Autodesk Inventor part; units mm, degrees
note: some values were not read from the file. Chosen so that the rebuilt part matches the saved one: direction of "Hole2".
(part 4 of 20)
  ellipse E392 centre (-10072.326927, -10029.332215) end of major axis (-10072.501043, -10029.408266) minor radius 0.168992 (-10072.321099, -10029.159944) -> (-10072.360635, -10029.165817) ccw
  ellipse E393 centre (-10070.302682, -10029.229876) end of major axis (-10070.476798, -10029.305926) minor radius 0.168992 (-10070.177973, -10029.092016) -> (-10070.296853, -10029.057605) ccw
  ellipse E394 centre (-10070.177499, -10030.249171) end of major axis (-10070.36739, -10030.242746) minor radius 0.079929 (-10070.142738, -10030.328755) -> (-10070.027446, -10030.302364) ccw
  ellipse E395 centre (-10072.201744, -10030.35151) end of major axis (-10072.391636, -10030.345086) minor radius 0.079929 (-10072.388447, -10030.360949) -> (-10072.166984, -10030.431094) ccw
  line L492 (-10072.72794, -10030.167115) -> (-10074.103641, -10030.236666)
  line L493 (-10074.255583, -10030.325688) -> (-10073.85675, -10031.238806)
  line L494 (-10067.96089, -10030.940729) -> (-10068.359722, -10030.027612)
  line L495 (-10068.581185, -10029.957468) -> (-10069.956886, -10030.027019)
  line L496 (-10072.723339, -10030.031111) -> (-10074.09904, -10030.100662)
  line L497 (-10068.576584, -10029.821464) -> (-10069.952284, -10029.891015)
  line L498 (-10067.956288, -10030.804726) -> (-10068.355121, -10029.891609)
  ellipse E396 centre (-10074.06888, -10030.316249) end of major axis (-10074.258772, -10030.309825) minor radius 0.079929 (-10074.103641, -10030.236666) -> (-10074.255583, -10030.325688) ccw
  ellipse E397 centre (-10068.546425, -10030.037051) end of major axis (-10068.356533, -10030.043476) minor radius 0.079929 (-10068.359722, -10030.027612) -> (-10068.581185, -10029.957468) ccw
  ellipse E398 centre (-10074.064279, -10030.180246) end of major axis (-10074.25417, -10030.173821) minor radius 0.079929 (-10074.09904, -10030.100662) -> (-10074.25417, -10030.173821) ccw
  ellipse E399 centre (-10068.541823, -10029.901048) end of major axis (-10068.351932, -10029.907472) minor radius 0.079929 (-10068.355121, -10029.891609) -> (-10068.576584, -10029.821464) ccw
  line L499 (-10074.258772, -10030.309825) -> (-10074.25417, -10030.173821)
  line L500 (-10067.871011, -10029.740777) -> (-10067.902882, -10030.682769)
  line L501 (-10067.875439, -10030.745598) -> (-10067.841392, -10029.73928)
  ellipse E400 centre (-10067.948619, -10030.578053) end of major axis (-10067.935996, -10030.827734) minor radius 0.044682 (-10067.956288, -10030.804726) -> (-10067.902882, -10030.682769) ccw
  ellipse E401 centre (-10073.84448, -10030.876129) end of major axis (-10073.824283, -10031.275619) minor radius 0.071491 (-10073.85675, -10031.238806) -> (-10073.824283, -10031.275619) ccw
  ellipse E402 centre (-10067.948619, -10030.578053) end of major axis (-10067.928422, -10030.977543) minor radius 0.071491 (-10067.96089, -10030.940729) -> (-10067.875439, -10030.745598) ccw
  line L502 (-10073.824283, -10031.275619) -> (-10072.075178, -10031.18719)
  line L503 (-10069.677528, -10031.065972) -> (-10067.928422, -10030.977543)
  ellipse E403 centre (-10072.802697, -10009.479709) end of major axis (-10072.614174, -10009.456065) minor radius 0.095931 (-10072.613936, -10009.458421) -> (-10072.809979, -10009.383969) ccw
  line L504 (-10072.614174, -10009.456065) -> (-10072.610843, -10009.482618)
  line L505 (-10072.598783, -10009.657643) -> (-10072.613936, -10009.458421)
  line L506 (-10070.180999, -10009.3015) -> (-10070.166094, -10009.497453)
  line L507 (-10070.347572, -10009.614481) -> (-10071.235682, -10009.714641)
  line L508 (-10072.809979, -10009.383969) -> (-10074.200844, -10009.540829)
  line L509 (-10074.382322, -10009.657857) -> (-10074.366628, -10009.864192)
  line L510 (-10068.337917, -10010.084094) -> (-10068.409482, -10009.143227)
  line L511 (-10068.326139, -10010.155581) -> (-10068.374133, -10009.524607)
  ellipse E404 centre (-10074.193562, -10009.636569) end of major axis (-10074.382085, -10009.660213) minor radius 0.095931 (-10074.200844, -10009.540829) -> (-10074.382322, -10009.657857) ccw
  ellipse E405 centre (-10070.354854, -10009.518741) end of major axis (-10070.166331, -10009.495097) minor radius 0.095931 (-10070.347572, -10009.614481) -> (-10070.166094, -10009.497453) ccw
  ellipse E406 centre (-10068.294951, -10010.426681) end of major axis (-10068.250123, -10010.824161) minor radius 0.00852 (-10068.337917, -10010.084094) -> (-10068.331861, -10010.154713) ccw
  line L512 (-10074.363014, -10028.330212) -> (-10074.369736, -10028.432806)
  line L513 (-10068.399185, -10028.956994) -> (-10068.349903, -10028.204791)
  line L514 (-10068.533523, -10028.105039) -> (-10068.666725, -10028.090017)
  line L515 (-10068.370793, -10028.641723) -> (-10068.333284, -10028.069217)
  line L516 (-10072.60135, -10028.632241) -> (-10072.595095, -10028.536769)
  line L517 (-10071.184925, -10028.471649) -> (-10070.345198, -10028.566352)
  line L518 (-10070.161579, -10028.666104) -> (-10070.177271, -10028.905625)
  ellipse E407 centre (-10072.557033, -10028.27071) end of major axis (-10072.60186, -10028.668191) minor radius 0.00852 (-10072.60135, -10028.632241) -> (-10072.602641, -10028.659347) ccw
  ellipse E408 centre (-10070.132954, -10028.544094) end of major axis (-10070.177781, -10028.941574) minor radius 0.00852 (-10070.177271, -10028.905625) -> (-10070.177781, -10028.941574) ccw
  ellipse E409 centre (-10070.350339, -10028.644816) end of major axis (-10070.16175, -10028.667933) minor radius 0.078528 (-10070.161579, -10028.666104) -> (-10070.345198, -10028.566352) ccw
  ellipse E410 centre (-10068.538663, -10028.183503) end of major axis (-10068.350075, -10028.206621) minor radius 0.078528 (-10068.349903, -10028.204791) -> (-10068.533523, -10028.105039) ccw
  ellipse E411 centre (-10068.522044, -10028.047929) end of major axis (-10068.333456, -10028.071046) minor radius 0.078528 (-10068.333284, -10028.069217) -> (-10068.343012, -10028.040958) ccw
  ellipse E412 centre (-10074.325419, -10028.071275) end of major axis (-10074.370246, -10028.468755) minor radius 0.00852 (-10074.369736, -10028.432806) -> (-10074.370246, -10028.468755) ccw
  line L519 (-10074.370246, -10028.468755) -> (-10074.342698, -10028.471862)
  line L520 (-10070.177781, -10028.941574) -> (-10070.167273, -10028.942759)
  ellipse E413 centre (-10072.246386, -10007.126413) end of major axis (-10072.067085, -10007.189273) minor radius 0.159857 (-10072.059684, -10007.135852) -> (-10072.10068, -10007.038353) ccw
  ellipse E414 centre (-10072.273208, -10007.202921) end of major axis (-10072.093908, -10007.265781) minor radius 0.159857 (-10072.086506, -10007.21236) -> (-10072.121744, -10007.121966) ccw
  ellipse E415 centre (-10072.289789, -10007.05931) end of major axis (-10072.100103, -10007.048406) minor radius 0.096916 (-10072.103087, -10007.068749) -> (-10072.100103, -10007.048406) ccw
  ellipse E416 centre (-10072.297194, -10006.930504) end of major axis (-10072.107507, -10006.9196) minor radius 0.096916 (-10072.110492, -10006.939943) -> (-10072.263219, -10006.833594) ccw
  ellipse E417 centre (-10069.52614, -10007.0706) end of major axis (-10069.715826, -10007.081504) minor radius 0.096916 (-10069.492164, -10006.97369) -> (-10069.712842, -10007.061161) ccw
  line L521 (-10072.107507, -10006.9196) -> (-10072.100103, -10007.048406)
  line L522 (-10072.081203, -10007.304616) -> (-10072.086506, -10007.21236)
  line L523 (-10072.059684, -10007.135852) -> (-10072.047289, -10007.35146)
  line L524 (-10072.221358, -10007.256177) -> (-10072.110492, -10006.939943)
  line L525 (-10072.103087, -10007.068749) -> (-10072.19317, -10007.3257)
  line L526 (-10072.500311, -10008.05186) -> (-10072.396598, -10007.756029)
  line L527 (-10072.17592, -10007.668558) -> (-10070.151675, -10007.770897)
  line L528 (-10069.998948, -10007.877247) -> (-10070.102661, -10008.173078)
  line L529 (-10069.712842, -10007.061161) -> (-10069.823708, -10007.377394)
  line L530 (-10070.044385, -10007.464865) -> (-10072.068631, -10007.362526)
  ellipse E418 centre (-10072.480566, -10008.395343) end of major axis (-10072.460369, -10007.995853) minor radius 0.071491 (-10072.500311, -10008.05186) -> (-10072.554705, -10008.484751) ccw
  ellipse E419 centre (-10072.480566, -10008.395343) end of major axis (-10072.493189, -10008.645024) minor radius 0.044682 (-10072.492906, -10008.180666) -> (-10072.525255, -10008.39437) ccw
  line L531 (-10072.389193, -10007.884835) -> (-10072.492906, -10008.180666)
  ellipse E420 centre (-10070.082916, -10008.51656) end of major axis (-10070.103113, -10008.91605) minor radius 0.071491 (-10070.102661, -10008.173078) -> (-10070.157073, -10008.608429) ccw
  line L532 (-10070.14427, -10007.899703) -> (-10072.168516, -10007.797364)
  line L533 (-10070.358201, -10009.301066) -> (-10070.663673, -10009.285622)
  line L534 (-10071.882761, -10009.223989) -> (-10072.312978, -10009.202239)
  line L535 (-10067.939751, -10007.422007) -> (-10067.880499, -10008.452725)
  line L536 (-10067.849188, -10008.454308) -> (-10067.912929, -10007.345499)
  ellipse E421 centre (-10068.126453, -10007.412568) end of major axis (-10067.947153, -10007.475428) minor radius 0.159857 (-10067.939751, -10007.422007) -> (-10067.974989, -10007.331613) ccw
  ellipse E422 centre (-10068.099631, -10007.33606) end of major axis (-10067.92033, -10007.39892) minor radius 0.159857 (-10067.912929, -10007.345499) -> (-10067.953925, -10007.248) ccw
  line L537 (-10072.263219, -10006.833594) -> (-10073.63892, -10006.764043)
  line L538 (-10073.859597, -10006.851514) -> (-10074.249416, -10007.963431)
  line L539 (-10068.353556, -10008.261507) -> (-10067.963737, -10007.14959)
  line L540 (-10068.116464, -10007.043241) -> (-10069.492164, -10006.97369)
  line L541 (-10068.346151, -10008.390313) -> (-10067.956332, -10007.278396)
  ellipse E423 centre (-10073.672895, -10006.860953) end of major axis (-10073.862581, -10006.871858) minor radius 0.096916 (-10073.63892, -10006.764043) -> (-10073.859597, -10006.851514) ccw
  ellipse E424 centre (-10068.150439, -10007.140151) end of major axis (-10067.960752, -10007.129247) minor radius 0.096916 (-10067.963737, -10007.14959) -> (-10068.116464, -10007.043241) ccw
  ellipse E425 centre (-10068.143034, -10007.268957) end of major axis (-10067.953347, -10007.258053) minor radius 0.096916 (-10067.956332, -10007.278396) -> (-10067.953347, -10007.258053) ccw
  line L542 (-10067.960752, -10007.129247) -> (-10067.953347, -10007.258053)
  ellipse E426 centre (-10072.209895, -10007.765468) end of major axis (-10072.399582, -10007.776372) minor radius 0.096916 (-10072.17592, -10007.668558) -> (-10072.396598, -10007.756029) ccw
  ellipse E427 centre (-10070.18565, -10007.867808) end of major axis (-10069.995963, -10007.856903) minor radius 0.096916 (-10069.998948, -10007.877247) -> (-10070.151675, -10007.770897) ccw
  ellipse E428 centre (-10070.01041, -10007.367955) end of major axis (-10069.820723, -10007.357051) minor radius 0.096916 (-10070.044385, -10007.464865) -> (-10069.823708, -10007.377394) ccw
  ellipse E429 centre (-10072.034655, -10007.265616) end of major axis (-10072.224342, -10007.27652) minor radius 0.096916 (-10072.221358, -10007.256177) -> (-10072.068631, -10007.362526) ccw
  ellipse E430 centre (-10072.202491, -10007.894274) end of major axis (-10072.392178, -10007.905178) minor radius 0.096916 (-10072.168516, -10007.797364) -> (-10072.389193, -10007.884835) ccw
  ellipse E431 centre (-10072.313886, -10008.961649) end of major axis (-10072.493186, -10008.898789) minor radius 0.159857 (-10072.33531, -10009.121035) -> (-10072.324798, -10009.122819) ccw
  ellipse E432 centre (-10072.340708, -10009.038157) end of major axis (-10072.161408, -10009.101016) minor radius 0.159857 (-10072.363459, -10009.197281) -> (-10072.348281, -10009.199785) ccw
  ellipse E433 centre (-10070.316463, -10009.140496) end of major axis (-10070.137162, -10009.203356) minor radius 0.159857 (-10070.251159, -10009.298888) -> (-10070.185446, -10009.268734) ccw
  ellipse E434 centre (-10070.28964, -10009.063988) end of major axis (-10070.468941, -10009.001128) minor radius 0.159857 (-10070.236148, -10009.224709) -> (-10070.189719, -10009.210719) ccw
  ellipse E435 centre (-10070.178245, -10007.996614) end of major axis (-10069.988559, -10007.985709) minor radius 0.096916 (-10070.019731, -10007.936529) -> (-10070.14427, -10007.899703) ccw
  line L543 (-10068.338763, -10009.424007) -> (-10068.374927, -10008.794905)
  line L544 (-10068.400279, -10008.897002) -> (-10068.388749, -10009.097559)
  line L545 (-10068.3686, -10009.448068) -> (-10068.365318, -10009.505168)
  ellipse E436 centre (-10068.33381, -10008.60499) end of major axis (-10068.321187, -10008.355308) minor radius 0.044682 (-10068.346151, -10008.390313) -> (-10068.371921, -10008.521801) ccw
  ellipse E437 centre (-10074.229671, -10008.306913) end of major axis (-10074.249868, -10008.706403) minor radius 0.071491 (-10074.249416, -10007.963431) -> (-10074.303499, -10008.450252) ccw
  ellipse E438 centre (-10068.33381, -10008.60499) end of major axis (-10068.354007, -10009.004479) minor radius 0.071491 (-10068.353556, -10008.261507) -> (-10068.4065, -10008.630689) ccw
  ellipse E439 centre (-10072.776909, -10029.133016) end of major axis (-10072.596108, -10029.074614) minor radius 0.167961 (-10072.789107, -10029.303177) -> (-10072.589277, -10029.13178) ccw
  ellipse E440 centre (-10072.755355, -10029.199743) end of major axis (-10072.574553, -10029.141341) minor radius 0.167961 (-10072.644451, -10029.32956) -> (-10072.567723, -10029.198507) ccw
  ellipse E441 centre (-10069.970499, -10029.181393) end of major axis (-10070.1513, -10029.239795) minor radius 0.167961 (-10070.1513, -10029.239795) -> (-10070.111114, -10029.303245) ccw
  ellipse E442 centre (-10072.761869, -10029.388593) end of major axis (-10072.572355, -10029.402178) minor radius 0.083645 (-10072.574237, -10029.387357) -> (-10072.789171, -10029.304073) ccw
  ellipse E443 centre (-10072.771499, -10029.522931) end of major axis (-10072.581985, -10029.536516) minor radius 0.083645 (-10072.583867, -10029.521695) -> (-10072.798801, -10029.43841) ccw
  ellipse E444 centre (-10069.986643, -10029.50458) end of major axis (-10070.176156, -10029.490995) minor radius 0.083645 (-10070.013945, -10029.42006) -> (-10070.174275, -10029.505817) ccw
  ellipse E445 centre (-10069.992053, -10029.114666) end of major axis (-10070.172854, -10029.173068) minor radius 0.167961 (-10070.179685, -10029.115902) -> (-10070.004251, -10029.284827) ccw
  ellipse E446 centre (-10069.977013, -10029.370243) end of major axis (-10070.166527, -10029.356658) minor radius 0.083645 (-10070.004315, -10029.285722) -> (-10070.166527, -10029.356658) ccw
  line L546 (-10070.172854, -10029.173068) -> (-10070.1513, -10029.239795)
  line L547 (-10070.166527, -10029.356658) -> (-10070.176156, -10029.490995)
  line L548 (-10072.531836, -10028.697875) -> (-10072.567723, -10029.198507)
  line L549 (-10072.589277, -10029.13178) -> (-10072.55339, -10028.631149)
  line L550 (-10072.494777, -10029.797499) -> (-10072.499038, -10029.784308)
  line L551 (-10072.49947, -10029.782969) -> (-10072.583867, -10029.521695)
  line L552 (-10072.574237, -10029.387357) -> (-10072.519259, -10029.557556)
  line L553 (-10070.174275, -10029.505817) -> (-10070.124475, -10029.659985)
  line L554 (-10070.245515, -10029.867378) -> (-10071.514069, -10029.875737)
  line L555 (-10071.955355, -10029.878645) -> (-10072.279843, -10029.880783)
  line L556 (-10070.161258, -10028.858843) -> (-10070.179685, -10029.115902)
  line L557 (-10072.270213, -10029.746445) -> (-10072.013835, -10029.744756)
  line L558 (-10070.580502, -10029.735311) -> (-10070.235885, -10029.73304)
  ellipse E447 centre (-10074.137908, -10029.208853) end of major axis (-10074.318709, -10029.267256) minor radius 0.167961 (-10074.318709, -10029.267256) -> (-10074.278523, -10029.330706) ccw
  ellipse E448 centre (-10068.587946, -10029.172282) end of major axis (-10068.407145, -10029.11388) minor radius 0.167961 (-10068.477042, -10029.3021) -> (-10068.400314, -10029.171046) ccw
  ellipse E449 centre (-10068.6095, -10029.105556) end of major axis (-10068.428699, -10029.047153) minor radius 0.167961 (-10068.621698, -10029.275716) -> (-10068.421868, -10029.104319) ccw
  ellipse E450 centre (-10074.159462, -10029.142127) end of major axis (-10074.340263, -10029.200529) minor radius 0.167961 (-10074.347094, -10029.143363) -> (-10074.171659, -10029.312287) ccw
  line L559 (-10074.318709, -10029.267256) -> (-10074.340263, -10029.200529)
  line L560 (-10068.400314, -10029.171046) -> (-10068.38691, -10028.984061)
  line L561 (-10068.368215, -10028.723256) -> (-10068.3415, -10028.350584)
  line L562 (-10068.621698, -10029.275716) -> (-10070.004251, -10029.284827)
  line L563 (-10068.409198, -10028.927568) -> (-10068.421868, -10029.104319)
  line L564 (-10074.347094, -10029.143363) -> (-10074.314985, -10028.695444)
  line L565 (-10072.789107, -10029.303177) -> (-10074.171659, -10029.312287)
  ellipse E451 centre (-10072.344204, -10028.696639) end of major axis (-10072.525005, -10028.755041) minor radius 0.167961 (-10072.437227, -10028.555214) -> (-10072.531836, -10028.697875) ccw
  ellipse E452 centre (-10070.272817, -10029.782857) end of major axis (-10070.083303, -10029.796442) minor radius 0.083645 (-10070.245515, -10029.867378) -> (-10070.155633, -10029.855516) ccw
  ellipse E453 centre (-10072.307144, -10029.796262) end of major axis (-10072.496658, -10029.782677) minor radius 0.083645 (-10072.494777, -10029.797499) -> (-10072.487277, -10029.812028) ccw
  ellipse E454 centre (-10072.307144, -10029.796262) end of major axis (-10072.117631, -10029.809847) minor radius 0.083645 (-10072.356839, -10029.874281) -> (-10072.279843, -10029.880783) ccw
  ellipse E455 centre (-10072.365758, -10028.629912) end of major axis (-10072.546559, -10028.688315) minor radius 0.167961 (-10072.539173, -10028.57563) -> (-10072.55339, -10028.631149) ccw
  ellipse E456 centre (-10070.263187, -10029.64852) end of major axis (-10070.452701, -10029.634935) minor radius 0.083645 (-10070.235885, -10029.73304) -> (-10070.172132, -10029.727297) ccw
  ellipse E457 centre (-10072.297515, -10029.661925) end of major axis (-10072.487028, -10029.64834) minor radius 0.083645 (-10072.347313, -10029.739925) -> (-10072.270213, -10029.746445) ccw
  line L566 (-10072.798801, -10029.43841) -> (-10074.181353, -10029.447521)
  line L567 (-10074.341684, -10029.533278) -> (-10074.268765, -10029.759019)
  line L568 (-10068.300338, -10029.853716) -> (-10068.416458, -10029.494234)
  line L569 (-10068.631392, -10029.41095) -> (-10070.013945, -10029.42006)
  line L570 (-10072.789171, -10029.304073) -> (-10074.171724, -10029.313183)
  line L571 (-10068.621762, -10029.276612) -> (-10070.004315, -10029.285722)
  line L572 (-10068.093576, -10030.329659) -> (-10068.406828, -10029.359896)
  ellipse E458 centre (-10074.154052, -10029.532041) end of major axis (-10074.343565, -10029.518456) minor radius 0.083645 (-10074.181353, -10029.447521) -> (-10074.341684, -10029.533278) ccw
  ellipse E459 centre (-10068.60409, -10029.49547) end of major axis (-10068.414576, -10029.509055) minor radius 0.083645 (-10068.416458, -10029.494234) -> (-10068.631392, -10029.41095) ccw
  ellipse E460 centre (-10074.144422, -10029.397704) end of major axis (-10074.333936, -10029.384119) minor radius 0.083645 (-10074.171724, -10029.313183) -> (-10074.333936, -10029.384119) ccw
  ellipse E461 centre (-10068.59446, -10029.361133) end of major axis (-10068.404946, -10029.374718) minor radius 0.083645 (-10068.406828, -10029.359896) -> (-10068.621762, -10029.276612) ccw
  line L573 (-10074.343565, -10029.518456) -> (-10074.333936, -10029.384119)
  line L574 (-10068.032803, -10030.094217) -> (-10068.041603, -10030.216974)
  line L575 (-10068.020049, -10030.283701) -> (-10068.004197, -10030.062566)
  ellipse E462 centre (-10068.077526, -10030.105763) end of major axis (-10068.075879, -10030.355758) minor radius 0.039312 (-10068.093576, -10030.329659) -> (-10068.041603, -10030.216974) ccw
  ellipse E463 centre (-10068.077526, -10030.105763) end of major axis (-10068.080162, -10029.705772) minor radius 0.062899 (-10068.046247, -10030.460713) -> (-10068.020049, -10030.283701) ccw
  line L576 (-10072.577571, -10009.532359) -> (-10072.577053, -10009.432226)
  line L577 (-10072.560025, -10009.540558) -> (-10072.560176, -10009.569905)
  line L578 (-10070.342414, -10009.407096) -> (-10072.389265, -10009.607054)
  ellipse E464 centre (-10074.155851, -10009.382773) end of major axis (-10074.344261, -10009.407304) minor radius 0.092496 (-10074.341028, -10009.382975) -> (-10074.344639, -10009.401215) ccw
  ellipse E465 centre (-10068.554808, -10008.967185) end of major axis (-10068.366398, -10008.942654) minor radius 0.092496 (-10068.366021, -10008.948742) -> (-10068.366398, -10008.942654) ccw
  line L579 (-10068.366462, -10008.942166) -> (-10068.366398, -10008.942654)
  line L580 (-10074.344639, -10009.401215) -> (-10074.344914, -10009.454519)
  line L581 (-10068.385879, -10009.388256) -> (-10068.384314, -10009.085206)
  line L582 (-10068.369231, -10009.57016) -> (-10068.367254, -10009.187466)
  line L583 (-10068.366026, -10008.949747) -> (-10068.366021, -10008.948742)
  ellipse E466 centre (-10070.341933, -10009.313958) end of major axis (-10070.153523, -10009.289427) minor radius 0.092496 (-10070.342414, -10009.407096) -> (-10070.179086, -10009.34494) ccw
  ellipse E467 centre (-10072.388783, -10009.513916) end of major axis (-10072.577193, -10009.538448) minor radius 0.092496 (-10072.577571, -10009.532359) -> (-10072.389265, -10009.607054) ccw
  line L584 (-10074.342817, -10028.466107) -> (-10074.337905, -10028.703084)
  line L585 (-10068.381381, -10029.035724) -> (-10068.386397, -10028.79374)
  line L586 (-10068.363977, -10028.927724) -> (-10068.369259, -10028.672848)
  line L587 (-10072.571652, -10028.760795) -> (-10072.574544, -10028.621296)
  line L588 (-10071.996094, -10028.594581) -> (-10070.340635, -10028.756304)
  line L589 (-10072.555629, -10028.586144) -> (-10072.554791, -10028.62657)
  ellipse E468 centre (-10072.385757, -10028.639739) end of major axis (-10072.574269, -10028.61601) minor radius 0.082693 (-10072.442527, -10028.554595) -> (-10072.574544, -10028.621296) ccw
  ellipse E469 centre (-10070.338906, -10028.839697) end of major axis (-10070.527419, -10028.815968) minor radius 0.082693 (-10070.171544, -10028.818209) -> (-10070.340635, -10028.756304) ccw
  ellipse E470 centre (-10074.292929, -10028.345775) end of major axis (-10074.33182, -10028.74388) minor radius 0.022991 (-10074.337905, -10028.703084) -> (-10074.33182, -10028.74388) ccw
  line L590 (-10074.33182, -10028.74388) -> (-10074.31855, -10028.745177)
  line L591 (-10068.066947, -10007.915921) -> (-10068.053326, -10008.079123)
  line L592 (-10068.026512, -10008.074856) -> (-10068.045991, -10007.841482)
  ellipse E471 centre (-10068.254579, -10007.914685) end of major axis (-10068.071689, -10007.966173) minor radius 0.162803 (-10068.066947, -10007.915921) -> (-10068.102794, -10007.828273) ccw
  ellipse E472 centre (-10068.233623, -10007.840246) end of major axis (-10068.050732, -10007.891735) minor radius 0.162803 (-10068.045991, -10007.841482) -> (-10068.063716, -10007.781657) ccw
  line L593 (-10072.569221, -10008.694112) -> (-10072.518848, -10008.515183)
  line L594 (-10072.274012, -10008.31323) -> (-10070.239685, -10008.326635)
  ellipse E473 centre (-10072.540238, -10009.041373) end of major axis (-10072.537602, -10008.641381) minor radius 0.062899 (-10072.569221, -10008.694112) -> (-10072.596122, -10009.239876) ccw
  line L595 (-10072.579374, -10009.440527) -> (-10072.596122, -10009.239876)
  line L596 (-10072.575165, -10009.165437) -> (-10072.540188, -10009.584505)
  ellipse E474 centre (-10072.540238, -10009.041373) end of major axis (-10072.541885, -10009.291367) minor radius 0.039312 (-10072.558353, -10008.824335) -> (-10072.575165, -10009.165437) ccw
  line L597 (-10072.512857, -10008.662732) -> (-10072.558353, -10008.824335)
  line L598 (-10070.18653, -10009.255753) -> (-10070.176942, -10009.370631)
  ellipse E475 centre (-10070.130646, -10009.05725) end of major axis (-10070.133281, -10009.457242) minor radius 0.062899 (-10070.169022, -10008.750397) -> (-10070.18653, -10009.255753) ccw
  line L599 (-10070.228816, -10008.456858) -> (-10070.680232, -10008.453883)
  line L600 (-10071.788331, -10008.446582) -> (-10072.263143, -10008.443453)
  ellipse E476 centre (-10072.300557, -10008.407519) end of major axis (-10072.489899, -10008.423323) minor radius 0.093287 (-10072.274012, -10008.31323) -> (-10072.354057, -10008.321175) ccw
  ellipse E477 centre (-10070.26623, -10008.420924) end of major axis (-10070.455571, -10008.436728) minor radius 0.093287 (-10070.138972, -10008.343573) -> (-10070.239685, -10008.326635) ccw
  ellipse E478 centre (-10072.289688, -10008.537742) end of major axis (-10072.100347, -10008.521939) minor radius 0.093287 (-10072.263143, -10008.443453) -> (-10072.322447, -10008.447689) ccw
  ellipse E479 centre (-10070.255361, -10008.551147) end of major axis (-10070.066019, -10008.535344) minor radius 0.093287 (-10070.216901, -10008.457129) -> (-10070.228816, -10008.456858) ccw
  ellipse E480 centre (-10070.255361, -10008.551147) end of major axis (-10070.066019, -10008.535344) minor radius 0.093287 (-10070.151471, -10008.466353) -> (-10070.195146, -10008.458654) ccw
  line L601 (-10068.401813, -10008.721573) -> (-10068.358663, -10008.568304)
  line L602 (-10068.390944, -10008.851796) -> (-10068.086375, -10007.769954)
  line L603 (-10074.353939, -10009.228293) -> (-10074.335797, -10009.445646)
  ellipse E481 centre (-10068.372829, -10009.068833) end of major axis (-10068.371181, -10008.818839) minor radius 0.039312 (-10068.390944, -10008.851796) -> (-10068.408326, -10009.185783) ccw
  ellipse E482 centre (-10074.298055, -10009.02979) end of major axis (-10074.30069, -10009.429781) minor radius 0.062899 (-10074.332168, -10008.702748) -> (-10074.353939, -10009.228293) ccw
  ellipse E483 centre (-10068.372829, -10009.068833) end of major axis (-10068.375464, -10009.468825) minor radius 0.062899 (-10068.401813, -10008.721573) -> (-10068.429051, -10009.263222) ccw
  ellipse E484 centre (-10068.274007, -10007.768718) end of major axis (-10068.084666, -10007.752915) minor radius 0.093287 (-10068.086375, -10007.769954) -> (-10068.084666, -10007.752915) ccw
  line L604 (-10068.089095, -10007.699848) -> (-10068.084666, -10007.752915)
  ellipse E485 centre (-10068.216608, -10029.12541) end of major axis (-10068.205462, -10029.56777) minor radius 0.074077 (-10068.281516, -10029.288259) -> (-10068.274706, -10029.351944) ccw
  ellipse E486 centre (-10068.255012, -10029.275153) end of major axis (-10068.25879, -10029.125201) minor radius 0.025111 (-10068.274706, -10029.351944) -> (-10068.261458, -10029.413159) ccw
  ellipse E487 centre (-10068.094104, -10029.659546) end of major axis (-10068.090325, -10029.809499) minor radius 0.025111 (-10068.100549, -10029.797552) -> (-10068.091278, -10029.809415) ccw
  ellipse E488 centre (-10068.08098, -10029.625954) end of major axis (-10068.077202, -10029.775906) minor radius 0.025111 (-10068.064626, -10029.753413) -> (-10068.063948, -10029.750531) ccw
  line L605 (-10068.100549, -10029.797552) -> (-10068.121454, -10029.747612)
  line L606 (-10068.164781, -10029.644109) -> (-10068.178644, -10029.610993)
  line L607 (-10068.250286, -10029.439846) -> (-10068.261458, -10029.413159)
  line L608 (-10068.176037, -10028.175225) -> (-10068.151259, -10028.234418)
  ellipse E489 centre (-10068.150709, -10028.956729) end of major axis (-10068.165318, -10028.376913) minor radius 0.097095 (-10068.247322, -10028.975539) -> (-10068.198058, -10029.418828) ccw
  ellipse E490 centre (-10068.234183, -10029.450753) end of major axis (-10068.241756, -10029.300944) minor radius 0.026809 (-10068.259943, -10029.468853) -> (-10068.259052, -10029.480298) ccw
  ellipse E491 centre (-10068.234183, -10029.450753) end of major axis (-10068.241756, -10029.300944) minor radius 0.026809 (-10068.261999, -10029.414966) -> (-10068.261887, -10029.424904) ccw
  ellipse E492 centre (-10068.224513, -10029.534928) end of major axis (-10068.232087, -10029.385119) minor radius 0.026809 (-10068.244423, -10029.60764) -> (-10068.229114, -10029.670932) ccw
  ellipse E493 centre (-10068.044673, -10029.946667) end of major axis (-10068.037099, -10030.096476) minor radius 0.026809 (-10068.049274, -10030.08267) -> (-10068.032192, -10030.093539) ccw
  ellipse E494 centre (-10068.031107, -10029.915689) end of major axis (-10068.023533, -10030.065497) minor radius 0.026809 (-10068.011669, -10030.046675) -> (-10068.003665, -10029.978518) ccw
  line L609 (-10068.051046, -10030.097181) -> (-10068.037099, -10030.096476)
  ellipse E495 centre (-10068.185687, -10029.393139) end of major axis (-10068.163344, -10029.835075) minor radius 0.079087 (-10068.259052, -10029.480298) -> (-10068.244423, -10029.60764) ccw
  ellipse E496 centre (-10068.069012, -10029.660266) end of major axis (-10068.046669, -10030.102201) minor radius 0.079087 (-10068.032192, -10030.093539) -> (-10068.011669, -10030.046675) ccw
  line L610 (-10068.049274, -10030.08267) -> (-10068.229114, -10029.670932)
  line L611 (-10067.995835, -10029.747088) -> (-10068.003665, -10029.978518)
  ellipse E497 centre (-10068.117568, -10029.237584) end of major axis (-10068.088282, -10029.816845) minor radius 0.103663 (-10068.222533, -10029.211406) -> (-10068.043942, -10029.74952) ccw
  ellipse E498 centre (-10068.042587, -10008.251265) end of major axis (-10068.050161, -10008.401074) minor radius 0.026809 (-10068.015764, -10008.174757) -> (-10068.025304, -10008.113484) ccw
  ellipse E499 centre (-10068.057077, -10008.229125) end of major axis (-10068.049503, -10008.079316) minor radius 0.026809 (-10068.047224, -10008.07999) -> (-10068.064481, -10008.100319) ccw
  ellipse E500 centre (-10068.232852, -10008.730505) end of major axis (-10068.225278, -10008.580697) minor radius 0.026809 (-10068.240257, -10008.601699) -> (-10068.25466, -10008.671676) ccw
  ellipse E501 centre (-10068.241073, -10008.817424) end of major axis (-10068.233499, -10008.667616) minor radius 0.026809 (-10068.268315, -10008.885499) -> (-10068.267895, -10008.893932) ccw
  line L612 (-10068.049503, -10008.079316) -> (-10068.067092, -10008.078427)
  ellipse E502 centre (-10068.076289, -10008.519938) end of major axis (-10068.053946, -10008.078002) minor radius 0.079087 (-10068.025304, -10008.113484) -> (-10068.047224, -10008.07999) ccw
  ellipse E503 centre (-10068.190328, -10008.845221) end of major axis (-10068.212671, -10009.287157) minor radius 0.079087 (-10068.25466, -10008.671676) -> (-10068.260492, -10008.723479) ccw
  line L613 (-10068.240257, -10008.601699) -> (-10068.064481, -10008.100319)
  line L614 (-10068.251636, -10009.176766) -> (-10068.251813, -10009.17369)
  line L615 (-10068.264197, -10008.958267) -> (-10068.267895, -10008.893932)
  line L616 (-10068.015764, -10008.174757) -> (-10068.000133, -10008.446677)
  ellipse E504 centre (-10068.117568, -10008.956397) end of major axis (-10068.088282, -10008.377137) minor radius 0.103663 (-10068.043942, -10008.444462) -> (-10068.222533, -10008.982575) ccw
  line L617 (-10068.071921, -10010.081174) -> (-10068.031336, -10009.960354)
  ellipse E505 centre (-10067.886187, -10010.569675) end of major axis (-10067.942011, -10009.992368) minor radius 0.148512 (-10067.928583, -10009.993399) -> (-10068.007789, -10010.074909) ccw
  line L618 (-10068.031808, -10028.233631) -> (-10068.083473, -10028.111679)
  ellipse E506 centre (-10067.886187, -10027.624306) end of major axis (-10067.942011, -10028.201614) minor radius 0.148512 (-10068.007789, -10028.119073) -> (-10067.928583, -10028.200582) ccw
  ellipse E507 centre (-10068.284196, -10028.94286) end of major axis (-10068.285184, -10028.792864) minor radius 0.023587 (-10068.30575, -10028.876134) -> (-10068.307279, -10028.968276) ccw
  ellipse E508 centre (-10068.279147, -10029.02798) end of major axis (-10068.280136, -10028.877983) minor radius 0.023587 (-10068.299642, -10029.097047) -> (-10068.288777, -10029.162318) ccw
  ellipse E509 centre (-10068.239183, -10028.8933) end of major axis (-10068.236267, -10029.33579) minor radius 0.069582 (-10068.307279, -10028.968276) -> (-10068.299642, -10029.097047) ccw
  line L619 (-10068.266229, -10029.232122) -> (-10068.288777, -10029.162318)
  line L620 (-10068.131241, -10028.107013) -> (-10068.090216, -10028.234016)
  line L621 (-10068.30575, -10028.876134) -> (-10068.249786, -10028.095432)
  ellipse E510 centre (-10068.172892, -10028.749572) end of major axis (-10068.176714, -10028.169584) minor radius 0.091204 (-10068.134335, -10028.234307) -> (-10068.219426, -10029.236049) ccw
  ellipse E511 centre (-10068.295635, -10009.917412) end of major axis (-10068.281051, -10010.066701) minor radius 0.008622 (-10068.304209, -10009.786542) -> (-10068.305313, -10009.781373) ccw
  ellipse E512 centre (-10068.295635, -10009.917412) end of major axis (-10068.281051, -10010.066701) minor radius 0.008622 (-10068.295256, -10009.843882) -> (-10068.295553, -10009.841609) ccw
  ellipse E513 centre (-10068.302958, -10009.893536) end of major axis (-10068.317542, -10009.744247) minor radius 0.008622 (-10068.31639, -10009.745252) -> (-10068.319875, -10009.763607) ccw
  line L622 (-10068.317542, -10009.744247) -> (-10068.34502, -10009.746931)
  ellipse E514 centre (-10068.276765, -10010.182688) end of major axis (-10068.319788, -10009.742285) minor radius 0.025434 (-10068.305313, -10009.781373) -> (-10068.31639, -10009.745252) ccw
  line L623 (-10068.321903, -10010.156223) -> (-10068.319875, -10009.763607)
  line L624 (-10068.295256, -10009.843882) -> (-10068.261943, -10010.099737)
  ellipse E515 centre (-10068.24161, -10010.615202) end of major axis (-10068.298002, -10010.03795) minor radius 0.033337 (-10068.27642, -10010.101151) -> (-10068.306562, -10010.158547) ccw
  line L625 (-10068.316409, -10028.42426) -> (-10068.324412, -10028.038139)
  line L626 (-10068.261141, -10028.094323) -> (-10068.290461, -10028.327252)
  ellipse E516 centre (-10068.299543, -10028.290269) end of major axis (-10068.314127, -10028.439558) minor radius 0.008622 (-10068.316409, -10028.42426) -> (-10068.312353, -10028.437292) ccw
  ellipse E517 centre (-10068.291825, -10028.261416) end of major axis (-10068.306409, -10028.410705) minor radius 0.008622 (-10068.300677, -10028.393642) -> (-10068.290461, -10028.327252) ccw
  line L627 (-10068.33142, -10028.437869) -> (-10068.314127, -10028.439558)
  ellipse E518 centre (-10068.274563, -10028.003575) end of major axis (-10068.317586, -10028.443978) minor radius 0.025434 (-10068.312353, -10028.437292) -> (-10068.300677, -10028.393642) ccw
  ellipse E519 centre (-10068.24161, -10027.578779) end of major axis (-10068.298002, -10028.156031) minor radius 0.033337 (-10068.306562, -10028.035434) -> (-10068.27642, -10028.09283) ccw
  line L628 (-10068.292643, -10009.076273) -> (-10068.242806, -10008.89925)
  line L629 (-10068.206906, -10008.771729) -> (-10068.204505, -10008.763202)
  line L630 (-10068.246022, -10010.098182) -> (-10068.307002, -10009.367577)
  line L631 (-10068.094635, -10009.959937) -> (-10068.130374, -10010.086884)
  ellipse E520 centre (-10068.281774, -10009.206496) end of major axis (-10068.280786, -10009.056499) minor radius 0.023587 (-10068.292643, -10009.076273) -> (-10068.302917, -10009.145302) ccw
  ellipse E521 centre (-10068.286045, -10009.293138) end of major axis (-10068.285057, -10009.143142) minor radius 0.023587 (-10068.309377, -10009.276377) -> (-10068.307002, -10009.367577) ccw
  ellipse E522 centre (-10068.240547, -10009.325823) end of major axis (-10068.243463, -10009.768314) minor radius 0.069582 (-10068.302917, -10009.145302) -> (-10068.309377, -10009.276377) ccw
  ellipse E523 centre (-10068.172892, -10009.44441) end of major axis (-10068.176714, -10010.024397) minor radius 0.091204 (-10068.219426, -10008.957933) -> (-10068.134335, -10009.959675) ccw
  line L632 (-10070.182233, -10029.678947) -> (-10070.171374, -10029.704889)
  line L633 (-10072.258497, -10029.746368) -> (-10072.264754, -10029.73142)
  line L634 (-10070.180085, -10029.632945) -> (-10070.169774, -10029.657578)
  line L635 (-10070.182233, -10029.678947) -> (-10070.282269, -10029.681468)
  ellipse E524 centre (-10070.323192, -10029.583707) end of major axis (-10070.57292, -10029.572043) minor radius 0.097367 (-10070.569586, -10029.589915) -> (-10070.282269, -10029.681468) ccw
  line L636 (-10070.569586, -10029.589915) -> (-10070.716026, -10029.240085)
  line L637 (-10070.830953, -10029.203464) -> (-10072.023499, -10029.233512)
  line L638 (-10072.105687, -10029.2751) -> (-10072.013016, -10029.496483)
  ellipse E525 centre (-10072.205641, -10029.631139) end of major axis (-10072.455369, -10029.619475) minor radius 0.097367 (-10072.164718, -10029.7289) -> (-10072.030137, -10029.707433) ccw
  line L639 (-10072.164718, -10029.7289) -> (-10072.264754, -10029.73142)
  line L640 (-10072.021351, -10029.18751) -> (-10070.828805, -10029.157462)
  line L641 (-10072.262605, -10029.685418) -> (-10072.162569, -10029.682898)
  ellipse E526 centre (-10072.203492, -10029.585137) end of major axis (-10071.953765, -10029.596801) minor radius 0.097367 (-10072.162569, -10029.682898) -> (-10072.047599, -10029.667455) ccw
  line L642 (-10070.713878, -10029.194083) -> (-10070.567438, -10029.543914)
  ellipse E527 centre (-10070.321044, -10029.537705) end of major axis (-10070.570771, -10029.526041) minor radius 0.097367 (-10070.567438, -10029.543914) -> (-10070.280121, -10029.635466) ccw
  line L643 (-10070.280121, -10029.635466) -> (-10070.180085, -10029.632945)
  line L644 (-10072.264754, -10029.73142) -> (-10072.262605, -10029.685418)
  line L645 (-10070.180085, -10029.632945) -> (-10070.182233, -10029.678947)
  ellipse E528 centre (-10070.814584, -10029.242568) end of major axis (-10070.714693, -10029.247233) minor radius 0.038947 (-10070.716026, -10029.240085) -> (-10070.830953, -10029.203464) ccw
  ellipse E529 centre (-10072.00713, -10029.272616) end of major axis (-10072.107021, -10029.267951) minor radius 0.038947 (-10072.023499, -10029.233512) -> (-10072.105687, -10029.2751) ccw
  ellipse E530 centre (-10070.812435, -10029.196566) end of major axis (-10070.712544, -10029.201231) minor radius 0.038947 (-10070.713878, -10029.194083) -> (-10070.828805, -10029.157462) ccw
  ellipse E531 centre (-10072.004981, -10029.226614) end of major axis (-10072.104872, -10029.221949) minor radius 0.038947 (-10072.021351, -10029.18751) -> (-10072.104872, -10029.221949) ccw
  line L646 (-10072.107021, -10029.267951) -> (-10072.104872, -10029.221949)
  line L647 (-10070.241901, -10009.179875) -> (-10070.237713, -10009.229762)
  line L648 (-10072.324422, -10009.127402) -> (-10072.322152, -10009.154438)
  line L649 (-10070.228286, -10009.223244) -> (-10070.234208, -10009.15271)
  ellipse E532 centre (-10070.508408, -10008.969253) end of major axis (-10070.748946, -10008.901127) minor radius 0.20633 (-10070.547072, -10009.172185) -> (-10070.435432, -10009.174998) ccw
  ellipse E533 centre (-10072.092227, -10008.929346) end of major axis (-10072.332766, -10008.861219) minor radius 0.20633 (-10072.130891, -10009.132278) -> (-10072.019251, -10009.135091) ccw
  spline S14 degree 3 poles (-10070.515578, -10008.746863) (-10070.5214, -10008.7475) (-10070.532983, -10008.748765) (-10070.550078, -10008.751995) (-10070.566778, -10008.756144) (-10070.583013, -10008.761269) (-10070.598727, -10008.767307) (-10070.61386, -10008.774226) (-10070.628351, -10008.781986) (-10070.642142, -10008.79055) (-10070.655173, -10008.79988) (-10070.667383, -10008.809937) (-10070.678715, -10008.820685) (-10070.689104, -10008.832086) (-10070.698501, -10008.844101) (-10070.706812, -10008.856703) (-10070.714092, -10008.869811) (-10070.71794, -10008.878985) (-10070.719859, -10008.883559) knots 0 0 0 0 0.0680148 0.13532856 0.20193874 0.26783312 0.33299287 0.39739576 0.46101961 0.52384586 0.58586341 0.64707277 0.70749045 0.76715357 0.82612483 0.88449738 0.9423997 1 1 1 1
  spline S15 degree 3 poles (-10070.712954, -10009.017327) (-10070.710929, -10009.021316) (-10070.706872, -10009.029309) (-10070.699756, -10009.040761) (-10070.691934, -10009.051805) (-10070.683371, -10009.062381) (-10070.674129, -10009.072477) (-10070.664245, -10009.082067) (-10070.653763, -10009.091129) (-10070.642724, -10009.099641) (-10070.63117, -10009.107578) (-10070.619143, -10009.114919) (-10070.606686, -10009.121641) (-10070.593839, -10009.127719) (-10070.580646, -10009.133136) (-10070.567144, -10009.137849) (-10070.553389, -10009.141905) (-10070.544051, -10009.143981) (-10070.539378, -10009.145021) knots 0 0 0 0 0.06018783 0.12057167 0.18123059 0.24222053 0.30357693 0.36531731 0.42744398 0.48994661 0.55280476 0.61599027 0.67946962 0.74320611 0.8071621 0.87130105 0.93558968 1 1 1 1
  spline S16 degree 3 poles (-10070.547072, -10009.172185) (-10070.551679, -10009.170991) (-10070.5609, -10009.1686) (-10070.574378, -10009.163772) (-10070.587555, -10009.158094) (-10070.600377, -10009.151521) (-10070.612823, -10009.144122) (-10070.624861, -10009.135936) (-10070.636463, -10009.127012) (-10070.647598, -10009.117394) (-10070.658237, -10009.107128) (-10070.668351, -10009.096258) (-10070.677911, -10009.084831) (-10070.686885, -10009.07289) (-10070.69525, -10009.060484) (-10070.702956, -10009.04765) (-10070.710042, -10009.034461) (-10070.714171, -10009.025383) (-10070.716235, -10009.020846) knots 0 0 0 0 0.06075211 0.12157744 0.18258462 0.24385247 0.30543277 0.36735321 0.42962038 0.49222284 0.55513405 0.61831518 0.68171776 0.7452863 0.80896074 0.87267882 0.93637843 1 1 1 1
  spline S17 degree 3 poles (-10070.738365, -10008.915545) (-10070.738051, -10008.908321) (-10070.737423, -10008.893872) (-10070.73369, -10008.872448) (-10070.727857, -10008.851688) (-10070.719885, -10008.831987) (-10070.710029, -10008.813658) (-10070.698444, -10008.796754) (-10070.685279, -10008.781271) (-10070.670679, -10008.767203) (-10070.654786, -10008.754542) (-10070.637742, -10008.743279) (-10070.619688, -10008.733407) (-10070.600762, -10008.724921) (-10070.581105, -10008.717805) (-10070.56085, -10008.712085) (-10070.540149, -10008.707633) (-10070.526126, -10008.705815) (-10070.519101, -10008.704905) knots 0 0 0 0 0.06486953 0.12974803 0.19473343 0.25817972 0.32016794 0.38123591 0.44183715 0.50233531 0.56300447 0.62403408 0.68553703 0.7475595 0.8100912 0.87307551 0.93641898 1 1 1 1
  spline S18 degree 3 poles (-10070.407011, -10008.707729) (-10070.400745, -10008.708979) (-10070.388387, -10008.711443) (-10070.370613, -10008.717248) (-10070.353844, -10008.72446) (-10070.338145, -10008.733155) (-10070.323548, -10008.743226) (-10070.310095, -10008.754612) (-10070.297823, -10008.767238) (-10070.28677, -10008.781035) (-10070.276973, -10008.795933) (-10070.26847, -10008.81186) (-10070.261297, -10008.828748) (-10070.255492, -10008.846526) (-10070.251084, -10008.865125) (-10070.248144, -10008.884475) (-10070.246579, -10008.904512) (-10070.246807, -10008.918072) (-10070.246922, -10008.924945) knots 0 0 0 0 0.06465055 0.1274876 0.18889307 0.24923877 0.30888211 0.36816237 0.42739777 0.48688361 0.54689159 0.60767024 0.6694463 0.73242683 0.79680187 0.8627473 0.93042784 1 1 1 1
  spline S19 degree 3 poles (-10070.269529, -10009.029389) (-10070.27154, -10009.034074) (-10070.275539, -10009.043389) (-10070.282439, -10009.056851) (-10070.289929, -10009.069795) (-10070.298053, -10009.082162) (-10070.306769, -10009.093931) (-10070.31606, -10009.105068) (-10070.3259, -10009.115546) (-10070.336269, -10009.125333) (-10070.347142, -10009.134401) (-10070.358496, -10009.142717) (-10070.370309, -10009.150254) (-10070.382557, -10009.156979) (-10070.395217, -10009.162868) (-10070.40827, -10009.167867) (-10070.421675, -10009.172034) (-10070.430837, -10009.174008) (-10070.435432, -10009.174998) knots 0 0 0 0 0.06647427 0.13218355 0.19716033 0.2614393 0.32505872 0.38806176 0.45049795 0.51242459 0.57390817 0.63502578 0.69586647 0.75653236 0.81713976 0.87781985 0.93871923 1 1 1 1
  spline S20 degree 3 poles (-10070.427738, -10009.147833) (-10070.424282, -10009.147222) (-10070.4174, -10009.146004) (-10070.407259, -10009.1435) (-10070.397329, -10009.140534) (-10070.387625, -10009.137074) (-10070.378153, -10009.133152) (-10070.365864, -10009.127336) (-10070.3511, -10009.118988) (-10070.334421, -10009.107402) (-10070.318887, -10009.094383) (-10070.304443, -10009.08017) (-10070.295862, -10009.069762) (-10070.291574, -10009.06456) knots 0 0 0 0 0.0644506 0.12832403 0.1917227 0.2547379 0.31744987 0.37992792 0.50437187 0.62845768 0.75238919 0.87624484 1 1 1 1
  spline S21 degree 3 poles (-10070.25127, -10008.850239) (-10070.252837, -10008.846758) (-10070.255949, -10008.839844) (-10070.261611, -10008.830032) (-10070.267923, -10008.82075) (-10070.274935, -10008.812027) (-10070.282603, -10008.803852) (-10070.290906, -10008.796227) (-10070.29982, -10008.789148) (-10070.309321, -10008.782613) (-10070.319383, -10008.776618) (-10070.329984, -10008.771161) (-10070.341099, -10008.76624) (-10070.352706, -10008.761853) (-10070.364779, -10008.757993) (-10070.377298, -10008.754671) (-10070.390232, -10008.751836) (-10070.399038, -10008.750409) (-10070.403489, -10008.749688) knots 0 0 0 0 0.05994656 0.11908522 0.17773662 0.23620436 0.29477068 0.35369309 0.41320222 0.47350071 0.53476324 0.59713734 0.66074485 0.72568383 0.79203056 0.85984183 0.92915698 1 1 1 1
  spline S22 degree 3 poles (-10072.099397, -10008.706956) (-10072.105804, -10008.707668) (-10072.118543, -10008.709083) (-10072.137307, -10008.712815) (-10072.155575, -10008.717652) (-10072.173259, -10008.723659) (-10072.190282, -10008.730753) (-10072.206562, -10008.738893) (-10072.222022, -10008.748024) (-10072.236582, -10008.758098) (-10072.250161, -10008.769064) (-10072.262681, -10008.780871) (-10072.274062, -10008.79347) (-10072.284219, -10008.806813) (-10072.293084, -10008.820846) (-10072.300534, -10008.83553) (-10072.306635, -10008.85078) (-10072.30937, -10008.86135) (-10072.310737, -10008.866637) knots 0 0 0 0 0.06847843 0.13617931 0.20309758 0.26921597 0.33450964 0.39895103 0.46251501 0.52518448 0.58695626 0.64784755 0.70790276 0.76720073 0.82586204 0.88405611 0.94200741 1 1 1 1
  spline S23 degree 3 poles (-10072.288058, -10008.993509) (-10072.285874, -10008.996992) (-10072.281494, -10009.003973) (-10072.274132, -10009.01395) (-10072.266216, -10009.023568) (-10072.25772, -10009.032771) (-10072.248692, -10009.041554) (-10072.239159, -10009.049896) (-10072.229156, -10009.05778) (-10072.218713, -10009.065188) (-10072.207863, -10009.072103) (-10072.196639, -10009.078507) (-10072.185071, -10009.084384) (-10072.173193, -10009.089713) (-10072.161037, -10009.094482) (-10072.148631, -10009.098658) (-10072.13602, -10009.10228) (-10072.127474, -10009.104168) (-10072.123197, -10009.105113) knots 0 0 0 0 0.06025982 0.1207868 0.18162334 0.24279657 0.30432017 0.36619627 0.42841724 0.49096745 0.55382495 0.61696316 0.68035239 0.74396143 0.807759 0.87171523 0.93580312 1 1 1 1
  spline S24 degree 3 poles (-10072.130891, -10009.132278) (-10072.135168, -10009.131176) (-10072.143726, -10009.128971) (-10072.156262, -10009.124591) (-10072.168542, -10009.119474) (-10072.180524, -10009.113577) (-10072.192189, -10009.106958) (-10072.203512, -10009.099648) (-10072.21447, -10009.091684) (-10072.225039, -10009.083103) (-10072.235197, -10009.073941) (-10072.244919, -10009.064234) (-10072.254182, -10009.054018) (-10072.262961, -10009.04333) (-10072.271237, -10009.032207) (-10072.278971, -10009.020679) (-10072.286193, -10009.008808) (-10072.290519, -10009.000618) (-10072.292681, -10008.996523) knots 0 0 0 0 0.06083705 0.12173396 0.18278727 0.24406937 0.30563053 0.36750102 0.4296934 0.49220474 0.55501884 0.61810841 0.68143706 0.74496132 0.80863248 0.87239845 0.9362055 1 1 1 1
  spline S25 degree 3 poles (-10072.32153, -10008.896639) (-10072.321902, -10008.888957) (-10072.322644, -10008.873619) (-10072.320757, -10008.850624) (-10072.316519, -10008.828006) (-10072.309731, -10008.80624) (-10072.30065, -10008.785762) (-10072.289501, -10008.766869) (-10072.276477, -10008.749579) (-10072.26175, -10008.733887) (-10072.245493, -10008.719783) (-10072.227876, -10008.707258) (-10072.209067, -10008.696301) (-10072.189232, -10008.686905) (-10072.168538, -10008.679052) (-10072.147144, -10008.67277) (-10072.125232, -10008.667914) (-10072.110368, -10008.665971) (-10072.10292, -10008.664997) knots 0 0 0 0 0.06491361 0.12961858 0.19438015 0.25897481 0.32176837 0.38321901 0.44389655 0.50426715 0.56468953 0.62541836 0.68661292 0.74834873 0.81063045 0.87340478 0.93657257 1 1 1 1
  spline S26 degree 3 poles (-10071.990831, -10008.667822) (-10071.984217, -10008.669151) (-10071.971183, -10008.671769) (-10071.952487, -10008.678048) (-10071.934918, -10008.68589) (-10071.918552, -10008.695376) (-10071.903428, -10008.70638) (-10071.889593, -10008.71883) (-10071.877091, -10008.732639) (-10071.865969, -10008.747724) (-10071.856268, -10008.764002) (-10071.848034, -10008.781389) (-10071.841308, -10008.799804) (-10071.836135, -10008.819165) (-10071.832552, -10008.83939) (-10071.830636, -10008.860394) (-10071.830291, -10008.882111) (-10071.831485, -10008.896738) (-10071.832091, -10008.904163) knots 0 0 0 0 0.06410082 0.12632292 0.18708858 0.24680768 0.30587245 0.36465307 0.42349429 0.48271369 0.54260125 0.60342049 0.66541057 0.72878933 0.79375677 0.86049868 0.92919035 1 1 1 1